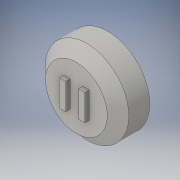
# Autodesk Inventor part: Dynamic Driver
Saved by Autodesk Inventor 2016 (Build 200138000, 138)
## iProperties
Created: 2015-07-24
Part Number: Dynamic Driver
Material: Generic
Document SubType Name: Modeling
Designer: Nancy
Density: 1 g/cm^3
Appearance: Default
Mass: 0.286193 g
Surface Area: 2.7078 cm^2
Volume: 0.286193 cm^3
Author: Nancy
Autodesk Inventor part; units mm, degrees
ref_plane "YZ Plane" through (0, 0, 0) normal (1, 0, 0) x (0, 1, 0)
ref_plane "XZ Plane" through (0, 0, 0) normal (0, 1, 0) x (-1, 0, 0)
sketch "Sketch3" plane through (0, 0, 0) normal (0, 0, 1) x (1, 0, 0)
  circle A0 centre (0, 0) radius 5.08
  dimension "d0" = 10.16
  constraints: 1 centre point, 1 coincident
  measures "d0" diameter of A0
extrude "Extrusion1" add sketch "Sketch3" along normal blind 2.54
ref_plane "Work Plane1" through (0, 0, 3.81) normal (0, 0, 1) x (1, 0, 0)
sketch "Sketch4" plane through (0, 0, 3.81) normal (0, 0, 1) x (1, 0, 0)
  circle A0 centre (0, 0) radius 3.7389
  dimension "d4" = 7.4778
  constraints: 1 centre point, 1 coincident
  measures "d4" diameter of A0
loft "Loft1" add profiles "Sketch4" section 2 edges at (-5.08, 0, 2.54)
sketch "Sketch5" plane through (0, 0, 3.81) normal (0, 0, 1) x (1, 0, 0)
  line L0 (-1.5443, -1.5992) -> (-0.7742, -1.5992)
  line L1 (-0.7742, -1.5992) -> (-0.7742, 1.5992)
  line L2 (-0.7742, 1.5992) -> (-1.5443, 1.5992)
  line L3 (-1.5443, 1.5992) -> (-1.5443, -1.5992)
  line L4 (0.7742, -1.5992) -> (1.5443, -1.5992)
  line L5 (1.5443, -1.5992) -> (1.5443, 1.5992)
  line L6 (1.5443, 1.5992) -> (0.7742, 1.5992)
  line L7 (0.7742, 1.5992) -> (0.7742, -1.5992)
  point P0 (0, 0)
  dimension "d9" = 0.7742
  dimension "d10" = 0.7742
  dimension "d11" = 1.5443
  dimension "d12" = 1.5443
  dimension "d23" = 1.5992
  dimension "d24" = 1.5992
  constraints: 16 end point, 4 parallel, 2 horizontal, 2 perpendicular, 2 point on line
  measures "d9" distance from line of point (0, 0) L1
  measures "d10" distance from line of L7 point (0, 0)
  measures "d11" distance from line of point (0, 0) L3
  measures "d12" distance from line of L5 point (0, 0)
  measures "d23" distance from line of point (0, 0) L2
  measures "d24" distance from line of L0 point (0, 0)
extrude "Extrusion2" add sketch "Sketch5" along normal blind 0.5161
sketch "Sketch6" plane through (-1.5443, -1.5992, 3.81) normal (0, -1, 0) x (1, 0, 0)
  circle A0 centre (0.384, 0.2581) radius 0.1676
  circle A1 centre (2.7046, 0.2581) radius 0.1676
  line L0 (0.7701, 0) -> (0.7701, 0.5161) projected
  line L1 (2.3185, 0) -> (2.3185, 0.5161) projected
  line L2 (-2.1946, 0) -> (5.2832, 0) projected
  point P0 (1.5443, -3.81)
  dimension "d15" = 0.3353
  dimension "d16" = 0.3353
  dimension "d17" = 0.3861
  dimension "d18" = 0.3861
  dimension "d25" = 0.2581
  dimension "d26" = 0.2581
  dimension "d27" = 0.5161
  constraints: 2 centre point
  measures "d15" diameter of A0
  measures "d16" diameter of A1
  measures "d17" distance from line of L0 A0.centre
  measures "d18" distance from line of A1.centre L1
  measures "d25" distance from line of L2 A0.centre
  measures "d26" distance from line of L2 A1.centre
  measures "d27" distance of L0.start L0.end
extrude "Extrusion3" cut sketch "Sketch6" against normal blind 2.54
equation "\"d4\" = 0.736 * d0"
equation "\"d9\" = 0.0762 * d0"
equation "\"d10\" = d9"
equation "\"d11\" = 0.152 * d0"
equation "\"d12\" = d11"
equation "\"d23\" = 0.1574 * d0"
equation "\"d24\" = d23"
equation "\"d13\" = 0.0508 * d0"
equation "\"d15\" = 0.033 * d0"
equation "\"d16\" = d15"
equation "\"d17\" = 0.038 * d0"
equation "\"d18\" = d17"
equation "\"d25\" = 0.5 * d27"
equation "\"d26\" = d25"
body "Solid1"
